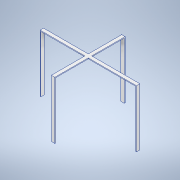
# Autodesk Inventor part: Soporte
Saved by Autodesk Inventor 2022.1 (Build 261234000, 234)
## iProperties
Created: 2021-10-03
Part Number: Soporte
Material: Aluminio 6061
Document SubType Name: Modeling
Designer: seb_0
Density: 2.7 g/cm^3
Appearance: Aluminio - Plano
Author: seb_0
Autodesk Inventor part; units mm, degrees
ref_plane "YZ Plane" through (0, 0, 0) normal (1, 0, 0) x (0, 1, 0)
ref_plane "XZ Plane" through (0, 0, 0) normal (0, 1, 0) x (-1, 0, 0)
ref_plane "XY Plane" through (0, 0, 0) normal (0, 0, 1) x (1, 0, 0)
sketch "Boceto1" plane through (0, 0, 0) normal (0, 1, 0) x (-1, 0, 0)
  line L0 (276.86, 5) -> (0, 5)
  line L1 (0, 5) -> (0, -5)
  line L2 (0, -5) -> (276.86, -5)
  line L3 (276.86, -5) -> (276.86, 5)
  line L4 (148.43, 100.33) -> (138.43, 100.33)
  line L5 (138.43, 100.33) -> (138.43, -100.33)
  line L6 (138.43, -100.33) -> (148.43, -100.33)
  line L7 (148.43, -100.33) -> (148.43, 100.33)
  line L8 (276.86, 0) -> (0, 0)
  point P0 (0, 0)
  point P1 (138.43, 0)
  point P2 (148.43, -5)
  point P3 (148.43, 5)
  point P4 (138.43, 5)
  point P5 (138.43, -5)
  dimension "d0" = 276.86
  dimension "d1" = 200.66
  dimension "d2" = 10
  dimension "d3" = 138.43
  constraints: 18 end point, 5 parallel, 4 midpoint, 3 perpendicular, 2 horizontal, 1 coincident
  measures "d0" distance of L0.start L0.end
  measures "d1" distance of L4.end L5.end
  measures "d2" distance of L2.end L0.start
  measures "d3" distance from line of point (0, 0) L5
extrude "Extrusión1" add sketch "Boceto1" along normal blind 2.5
sketch "Boceto2" plane through (-148.43, 0, 100.33) normal (0, 0, 1) x (1, 0, 0)
  line L0 (0, 0) -> (10, 0) projected
  line L1 (10, 0) -> (10, 2.5) projected
  line L2 (0, 2.5) -> (10, 2.5) projected
  line L3 (0, 0) -> (0, 2.5) projected
  line L4 (0, 0) -> (0, 2.5) projected
  line L5 (0, 0) -> (0, -165.1)
  line L6 (0, -165.1) -> (10, -165.1)
  line L7 (0, 0) -> (10, 0) projected
  line L8 (10, -165.1) -> (10, 0)
  point P0 (148.43, 0)
  dimension "d7" = 165.1
  constraints: 6 end point, 2 perpendicular, 1 vertical
  measures "d7" distance of L6.end L0.end
extrude "Extrusión2" add sketch "Boceto2" along normal blind 2.5
sketch "Boceto3" plane through (-138.43, 0, -100.33) normal (0, 0, -1) x (-1, 0, 0)
  line L0 (0, 0) -> (10, 0) projected
  line L1 (10, 0) -> (10, 2.5) projected
  line L2 (0, 2.5) -> (10, 2.5) projected
  line L3 (0, 0) -> (0, 2.5) projected
  line L4 (10, 0) -> (0, 0) projected
  line L5 (0, -165.1) -> (0, 0) projected
  line L6 (10, -165.1) -> (0, -165.1) projected
  line L7 (10, 0) -> (10, -165.1) projected
  point P0 (-138.43, 0)
extrude "Extrusión3" add sketch "Boceto3" along normal blind 2.5
sketch "Boceto4" plane through (0, 0, 5) normal (1, 0, 0) x (0, 0, -1)
  line L0 (0, 0) -> (10, 0) projected
  line L1 (10, 0) -> (10, 2.5) projected
  line L2 (0, 2.5) -> (10, 2.5) projected
  line L3 (0, 0) -> (0, 2.5) projected
  line L4 (0, 0) -> (0, -165.1)
  line L5 (0, -165.1) -> (10, -165.1)
  line L6 (10, -165.1) -> (10, 0)
  line L7 (105.33, 0) -> (105.33, -165.1) projected
  point P0 (5, 0)
  constraints: 6 end point, 2 perpendicular, 1 parallel, 1 vertical
extrude "Extrusión4" add sketch "Boceto4" along normal blind 2.5
sketch "Boceto5" plane through (-276.86, 0, -5) normal (-1, 0, 0) x (0, 0, 1)
  line L0 (0, 0) -> (10, 0) projected
  line L1 (10, 0) -> (10, 2.5) projected
  line L2 (0, 2.5) -> (10, 2.5) projected
  line L3 (0, 0) -> (0, 2.5) projected
  line L4 (10, 0) -> (0, 0) projected
  line L5 (0, -165.1) -> (0, 0) projected
  line L6 (10, -165.1) -> (0, -165.1) projected
  line L7 (10, 0) -> (10, -165.1) projected
  point P0 (5, 0)
extrude "Extrusión5" add sketch "Boceto5" along normal blind 2.5
